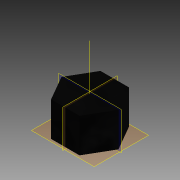
# Autodesk Inventor part: servo_metal_600TVL_shaft_nut
Saved by Autodesk Inventor 2015 SP1 (Build 190203100, 203)
## iProperties
Created: 2015-07-09
Part Number: servo_metal_600TVL_shaft_nut
Material: Generic
Document SubType Name: Modeling
Designer: Alexandre Cherpillod
Density: 1 g/cm^3
Appearance: Default
Author: Alexandre Cherpillod
Autodesk Inventor part; units mm, degrees
sketch "Sketch1" plane through (0, 0, 0) normal (0, 0, 1) x (1, 0, 0)
  line L0 (1.8764, 3.25) -> (3.7528, 0)
  line L1 (3.7528, 0) -> (1.8764, -3.25)
  line L2 (1.8764, -3.25) -> (-1.8764, -3.25)
  line L3 (-1.8764, -3.25) -> (-3.7528, 0)
  line L4 (-3.7528, 0) -> (-1.8764, 3.25)
  line L5 (-1.8764, 3.25) -> (1.8764, 3.25)
  point P0 (0, 0)
  point P1 (0, 0)
  dimension "d0" = 6.5
  constraints: 12 end point, 1 coincident, 1 horizontal, 13 other
  measures "d0" distance between parallel lines of L2 L5
extrude "Extrusion1" add sketch "Sketch1" along normal blind 4.5
body "Solid1"
